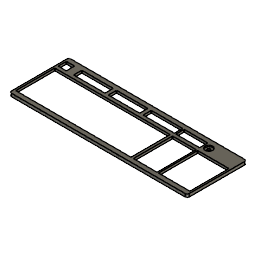
Top (Autodesk Fusion 360 design; units mm, degrees)
part number: 2026-01-27-17-33-11-118
Autodesk Fusion 360 part; units mm, degrees
(part 1 of 7)
sketch "Sketch1" plane through (0, 0, 0) normal (0, 0, 1) x (1, 0, 0)
  line L0 (-144.7637, -15.9426) -> (-144.7637, -18.7426)
  line L1 (-163.6637, -18.7426) -> (-163.6637, -15.9426)
  line L2 (-164.1637, -15.9426) -> (-164.1637, -18.7426)
  circle A0 centre (-169.0689, -18.2426) radius 2
  arc A1 (-107.101, -15.9426) -> (-108.601, -14.4426) centre (-108.601, -15.9426) ccw
  line L3 (-163.6635, 118.9832) -> (-163.6635, 116.1832)
  line L4 (-147.2637, -21.2426) -> (-161.6637, -21.2426)
  circle A2 centre (-169.0689, 118.4832) radius 2
  circle A3 centre (-169.0689, 118.4832) radius 1.7
  line L5 (-107.101, -15.9426) -> (-107.101, -18.7426)
  arc A4 (-144.7635, 116.1832) -> (-143.2635, 114.6832) centre (-143.2635, 116.1832) ccw
  arc A5 (-147.2637, -21.2426) -> (-144.7637, -18.7426) centre (-147.2637, -18.7426) ccw
  line L6 (-171.0689, 114.1832) -> (-165.6635, 114.1832)
  circle A6 centre (-151.9635, 117.5832) radius 1.7
  arc A7 (-164.1637, -18.7426) -> (-161.6637, -21.2426) centre (-161.6637, -18.7426) ccw
  line L7 (-161.6637, -20.7426) -> (-147.2637, -20.7426)
  circle A8 centre (-151.9635, 117.5832) radius 2
  line L8 (-165.6637, -13.9426) -> (-171.0689, -13.9426)
  circle A9 centre (-151.9637, -17.3426) radius 1.7
  line L9 (-165.6635, 114.6832) -> (-171.5689, 114.6832)
  arc A10 (-107.101, -18.7426) -> (-104.601, -21.2426) centre (-104.601, -18.7426) ccw
  arc A11 (-161.6635, 121.4832) -> (-164.1635, 118.9832) centre (-161.6635, 118.9832) ccw
  line L10 (-164.1635, 116.1832) -> (-164.1635, 118.9832)
  line L11 (-171.5689, -14.4426) -> (-165.6637, -14.4426)
  line L12 (-144.7635, 116.1832) -> (-144.7635, 118.9832)
  arc A12 (-169.0689, 123.4832) -> (-174.0689, 118.4832) centre (-169.0689, 118.4832) ccw
  arc A13 (-174.0689, -18.2426) -> (-169.0689, -23.2426) centre (-169.0689, -18.2426) ccw
  arc A14 (-165.6635, 114.6832) -> (-164.1635, 116.1832) centre (-165.6635, 116.1832) ccw
  circle A15 centre (-94.901, -17.3426) radius 1.7
  circle A16 centre (-94.901, -17.3426) radius 2
  circle A17 centre (-169.0689, -18.2426) radius 1.7
  line L13 (-106.601, -18.7426) -> (-106.601, -15.9426)
  line L14 (-145.2635, 118.9832) -> (-145.2635, 116.1832)
  line L15 (-143.2637, -14.4426) -> (-108.601, -14.4426)
  arc A18 (-144.7635, 118.9832) -> (-147.2635, 121.4832) centre (-147.2635, 118.9832) ccw
  line L16 (-82.701, -15.9426) -> (-82.701, -18.7426)
  arc A19 (-85.201, -21.2426) -> (-82.701, -18.7426) centre (-85.201, -18.7426) ccw
  circle A20 centre (42.9656, 118.4832) radius 1.7
  line L17 (-145.2637, -18.7426) -> (-145.2637, -15.9426)
  line L18 (28.798, 120.9832) -> (9.398, 120.9832)
  line L19 (-174.0689, 118.4832) -> (-174.0689, -18.2426)
  line L20 (-83.201, -18.7426) -> (-83.201, -15.9426)
  line L21 (-171.0689, 108.1832) -> (-171.0689, -7.9426)
  arc A21 (-82.701, 116.1832) -> (-81.201, 114.6832) centre (-81.201, 116.1832) ccw
  line L22 (9.398, 121.4832) -> (28.798, 121.4832)
  line L23 (30.798, 118.9832) -> (30.798, 116.1832)
  line L24 (-108.601, 114.6832) -> (-143.2635, 114.6832)
  arc A22 (-81.201, -14.4426) -> (-82.701, -15.9426) centre (-81.201, -15.9426) ccw
  circle A23 centre (-94.901, 117.5832) radius 2
  arc A24 (-82.701, 118.9832) -> (-85.201, 121.4832) centre (-85.201, 118.9832) ccw
  circle A25 centre (19.098, 117.5832) radius 2
  line L25 (-82.701, 116.1832) -> (-82.701, 118.9832)
  line L26 (-107.101, 116.1832) -> (-107.101, 118.9832)
  line L27 (31.298, 116.1832) -> (31.298, 118.9832)
  circle A26 centre (-94.901, 117.5832) radius 1.7
  arc A27 (5.398, 114.6832) -> (6.898, 116.1832) centre (5.398, 116.1832) ccw
  arc A28 (-164.1637, -15.9426) -> (-165.6637, -14.4426) centre (-165.6637, -15.9426) ccw
  arc A29 (31.298, 116.1832) -> (32.798, 114.6832) centre (32.798, 116.1832) ccw
  line L28 (-83.201, 118.9832) -> (-83.201, 116.1832)
  line L29 (6.898, 116.1832) -> (6.898, 118.9832)
  circle A30 centre (19.098, 117.5832) radius 1.7
  arc A31 (31.298, 118.9832) -> (28.798, 121.4832) centre (28.798, 118.9832) ccw
  arc A32 (9.398, 121.4832) -> (6.898, 118.9832) centre (9.398, 118.9832) ccw
  circle A33 centre (-151.9637, -17.3426) radius 2
  line L30 (-106.601, 118.9832) -> (-106.601, 116.1832)
  line L31 (7.398, 118.9832) -> (7.398, 116.1832)
  line L32 (-158.7961, 123.4832) -> (-169.0689, 123.4832)
  line L33 (-161.6635, 121.4832) -> (-147.2635, 121.4832)
  arc A34 (-108.601, 114.6832) -> (-107.101, 116.1832) centre (-108.601, 116.1832) ccw
  line L34 (-147.2635, 120.9832) -> (-161.6635, 120.9832)
  arc A35 (-143.2637, -14.4426) -> (-144.7637, -15.9426) centre (-143.2637, -15.9426) ccw
  arc A36 (-104.601, 121.4832) -> (-107.101, 118.9832) centre (-104.601, 118.9832) ccw
  circle A37 centre (19.098, -17.3426) radius 1.7
  line L35 (262.156, 114.6832) -> (262.156, -14.4426)
  line L36 (-104.601, 121.4832) -> (-85.201, 121.4832)
  line L37 (184.173, -15.9426) -> (184.173, -18.7426)
  line L38 (185.673, -14.4426) -> (222.567, -14.4426)
  line L39 (113.674, -14.4426) -> (158.273, -14.4426)
  line L40 (158.273, 114.6832) -> (113.674, 114.6832)
  line L41 (248.467, -15.9426) -> (248.467, -18.7426)
  line L42 (264.656, -18.2426) -> (264.656, 118.4832)
  circle A38 centre (19.098, -17.3426) radius 2
  line L43 (245.967, -21.2426) -> (226.567, -21.2426)
  line L44 (183.673, -18.7426) -> (183.673, -15.9426)
  circle A39 centre (171.973, -17.3426) radius 1.7
  line L45 (-85.201, 120.9832) -> (-104.601, 120.9832)
  arc A40 (224.067, -18.7426) -> (226.567, -21.2426) centre (226.567, -18.7426) ccw
  line L46 (-171.5689, 114.6832) -> (-171.5689, -14.4426)
  line L47 (261.656, 114.1832) -> (261.656, -13.9426)
  arc A41 (159.773, -15.9426) -> (158.273, -14.4426) centre (158.273, -15.9426) ccw
  line L48 (-169.0689, -23.2426) -> (42.9656, -23.2426)
  line L49 (6.898, -15.9426) -> (6.898, -18.7426)
  arc A42 (6.898, -15.9426) -> (5.398, -14.4426) centre (5.398, -15.9426) ccw
  line L50 (7.398, -18.7426) -> (7.398, -15.9426)
  line L51 (5.398, 114.6832) -> (-81.201, 114.6832)
  line L52 (9.398, -20.7426) -> (28.798, -20.7426)
  arc A43 (6.898, -18.7426) -> (9.398, -21.2426) centre (9.398, -18.7426) ccw
  line L53 (-81.201, -14.4426) -> (5.398, -14.4426)
  line L54 (28.798, -21.2426) -> (9.398, -21.2426)
  line L55 (-171.0689, -13.9426) -> (-171.0689, 114.1832)
  arc A44 (264.656, 118.4832) -> (259.656, 123.4832) centre (259.656, 118.4832) ccw
  line L56 (181.673, 120.9832) -> (162.273, 120.9832)
  line L57 (248.467, 118.9832) -> (248.467, 116.1832)
  circle A45 centre (259.656, -18.2426) radius 2
  line L58 (226.567, -20.7426) -> (245.967, -20.7426)
  arc A46 (159.773, -18.7426) -> (162.273, -21.2426) centre (162.273, -18.7426) ccw
  circle A47 centre (236.267, -17.3426) radius 1.7
  line L59 (181.673, -21.2426) -> (162.273, -21.2426)
  circle A48 centre (236.267, -17.3426) radius 2
  line L60 (160.273, -18.7426) -> (160.273, -15.9426)
  arc A49 (245.967, -21.2426) -> (248.467, -18.7426) centre (245.967, -18.7426) ccw
  arc A50 (224.067, -15.9426) -> (222.567, -14.4426) centre (222.567, -15.9426) ccw
  arc A51 (181.673, -21.2426) -> (184.173, -18.7426) centre (181.673, -18.7426) ccw
  line L61 (224.567, -18.7426) -> (224.567, -15.9426)
  line L62 (247.967, -18.7426) -> (247.967, -15.9426)
  line L63 (159.773, -15.9426) -> (159.773, -18.7426)
  arc A52 (259.656, -23.2426) -> (264.656, -18.2426) centre (259.656, -18.2426) ccw
  line L64 (224.067, -15.9426) -> (224.067, -18.7426)
  circle A53 centre (259.656, -18.2426) radius 1.7
  line L65 (-85.201, -21.2426) -> (-104.601, -21.2426)
  circle A54 centre (171.973, -17.3426) radius 2
  arc A55 (32.798, -14.4426) -> (31.298, -15.9426) centre (32.798, -15.9426) ccw
  line L66 (162.273, -20.7426) -> (181.673, -20.7426)
  line L67 (31.298, -15.9426) -> (31.298, -18.7426)
  circle A56 centre (42.9656, -18.2426) radius 1.7
  arc A57 (28.798, -21.2426) -> (31.298, -18.7426) centre (28.798, -18.7426) ccw
  arc A58 (249.967, -14.4426) -> (248.467, -15.9426) centre (249.967, -15.9426) ccw
  line L68 (30.798, -18.7426) -> (30.798, -15.9426)
  arc A59 (185.673, -14.4426) -> (184.173, -15.9426) centre (185.673, -15.9426) ccw
  line L69 (-104.601, -20.7426) -> (-85.201, -20.7426)
  line L70 (249.967, -14.4426) -> (262.156, -14.4426)
  circle A60 centre (99.974, -17.3426) radius 1.7
  circle A61 centre (99.974, 117.5832) radius 2
  line L71 (88.274, -18.7426) -> (88.274, -15.9426)
  line L72 (109.674, -21.2426) -> (90.274, -21.2426)
  line L73 (87.774, -15.9426) -> (87.774, -18.7426)
  line L74 (87.774, 116.1832) -> (87.774, 118.9832)
  line L75 (112.174, 116.1832) -> (112.174, 118.9832)
  arc A62 (109.674, -21.2426) -> (112.174, -18.7426) centre (109.674, -18.7426) ccw
  arc A63 (112.174, 118.9832) -> (109.674, 121.4832) centre (109.674, 118.9832) ccw
  line L76 (111.674, -18.7426) -> (111.674, -15.9426)
  line L77 (90.274, 121.4832) -> (109.674, 121.4832)
  arc A64 (87.774, -18.7426) -> (90.274, -21.2426) centre (90.274, -18.7426) ccw
  arc A65 (90.274, 121.4832) -> (87.774, 118.9832) centre (90.274, 118.9832) ccw
  circle A66 centre (99.974, 117.5832) radius 1.7
  line L78 (259.656, 123.4832) -> (-158.7961, 123.4832)
  arc A67 (113.674, -14.4426) -> (112.174, -15.9426) centre (113.674, -15.9426) ccw
  line L79 (111.674, 118.9832) -> (111.674, 116.1832)
  line L80 (90.274, -20.7426) -> (109.674, -20.7426)
  line L81 (109.674, 120.9832) -> (90.274, 120.9832)
  line L82 (86.274, 114.6832) -> (32.798, 114.6832)
  arc A68 (112.174, 116.1832) -> (113.674, 114.6832) centre (113.674, 116.1832) ccw
  arc A69 (86.274, 114.6832) -> (87.774, 116.1832) centre (86.274, 116.1832) ccw
  line L83 (88.274, 118.9832) -> (88.274, 116.1832)
  line L84 (112.174, -15.9426) -> (112.174, -18.7426)
  circle A70 centre (99.974, -17.3426) radius 2
  arc A71 (87.774, -15.9426) -> (86.274, -14.4426) centre (86.274, -15.9426) ccw
  circle A72 centre (236.267, 117.5832) radius 1.7
  arc A73 (226.567, 121.4832) -> (224.067, 118.9832) centre (226.567, 118.9832) ccw
  line L85 (245.967, 120.9832) -> (226.567, 120.9832)
  line L86 (262.156, 114.6832) -> (249.967, 114.6832)
  circle A74 centre (236.267, 117.5832) radius 2
  arc A75 (184.173, 116.1832) -> (185.673, 114.6832) centre (185.673, 116.1832) ccw
  line L87 (224.067, 116.1832) -> (224.067, 118.9832)
  line L88 (226.567, 121.4832) -> (245.967, 121.4832)
  line L89 (-169.0689, -23.2426) -> (259.656, -23.2426)
  arc A76 (222.567, 114.6832) -> (224.067, 116.1832) centre (222.567, 116.1832) ccw
  line L90 (262.156, -14.4426) -> (-171.5689, -14.4426)
  line L91 (32.798, -14.4426) -> (86.274, -14.4426)
  line L92 (261.656, -7.9426) -> (261.656, 108.1832)
  line L93 (159.773, 116.1832) -> (159.773, 118.9832)
  line L94 (160.273, 118.9832) -> (160.273, 116.1832)
  arc A77 (248.467, 116.1832) -> (249.967, 114.6832) centre (249.967, 116.1832) ccw
  circle A78 centre (259.656, 118.4832) radius 1.7
  line L95 (-171.5689, 114.6832) -> (262.156, 114.6832)
  circle A79 centre (259.656, 118.4832) radius 2
  arc A80 (248.467, 118.9832) -> (245.967, 121.4832) centre (245.967, 118.9832) ccw
  arc A81 (158.273, 114.6832) -> (159.773, 116.1832) centre (158.273, 116.1832) ccw
  arc A82 (184.173, 118.9832) -> (181.673, 121.4832) centre (181.673, 118.9832) ccw
  line L96 (222.567, 114.6832) -> (185.673, 114.6832)
  line L97 (247.967, 118.9832) -> (247.967, 116.1832)
  line L98 (224.567, 118.9832) -> (224.567, 116.1832)
  line L99 (184.173, 116.1832) -> (184.173, 118.9832)
  line L100 (162.273, 121.4832) -> (181.673, 121.4832)
  circle A83 centre (171.973, 117.5832) radius 1.7
  circle A84 centre (171.973, 117.5832) radius 2
  line L101 (183.673, 118.9832) -> (183.673, 116.1832)
  arc A85 (162.273, 121.4832) -> (159.773, 118.9832) centre (162.273, 118.9832) ccw
  line L102 (-154.9635, 117.5832) -> (-154.9635, 114.6832)
  line L103 (-148.9635, 117.5832) -> (-148.9635, 114.6832)
  arc A86 (-148.9635, 117.5832) -> (-154.9635, 117.5832) centre (-151.9635, 117.5832) ccw
  line L104 (-97.901, 117.5832) -> (-97.901, 114.6832)
  arc A87 (-91.901, 117.5832) -> (-97.901, 117.5832) centre (-94.901, 117.5832) ccw
  line L105 (-91.901, 117.5832) -> (-91.901, 114.6832)
  line L106 (16.098, 117.5832) -> (16.098, 114.6832)
  arc A88 (22.098, 117.5832) -> (16.098, 117.5832) centre (19.098, 117.5832) ccw
  line L107 (22.098, 117.5832) -> (22.098, 114.6832)
  line L108 (102.974, 117.5832) -> (102.974, 114.6832)
  arc A89 (102.974, 117.5832) -> (96.974, 117.5832) centre (99.974, 117.5832) ccw
  line L109 (96.974, 117.5832) -> (96.974, 114.6832)
  line L110 (174.973, 117.5832) -> (174.973, 114.6832)
  arc A90 (174.973, 117.5832) -> (168.973, 117.5832) centre (171.973, 117.5832) ccw
  line L111 (168.973, 117.5832) -> (168.973, 114.6832)
  line L112 (239.267, 117.5832) -> (239.267, 114.6832)
  arc A91 (239.267, 117.5832) -> (233.267, 117.5832) centre (236.267, 117.5832) ccw
  line L113 (233.267, 117.5832) -> (233.267, 114.6832)
  line L114 (239.267, -17.3426) -> (239.267, -14.4426)
  arc A92 (233.267, -17.3426) -> (239.267, -17.3426) centre (236.267, -17.3426) ccw
  line L115 (233.267, -17.3426) -> (233.267, -14.4426)
  arc A93 (168.973, -17.3426) -> (174.973, -17.3426) centre (171.973, -17.3426) ccw
  line L116 (174.973, -17.3426) -> (174.973, -14.4426)
  line L117 (168.973, -17.3426) -> (168.973, -14.4426)
  line L118 (102.974, -17.3426) -> (102.974, -14.4426)
  arc A94 (96.974, -17.3426) -> (102.974, -17.3426) centre (99.974, -17.3426) ccw
  line L119 (96.974, -17.3426) -> (96.974, -14.4426)
  line L120 (22.098, -17.3426) -> (22.098, -14.4426)
  arc A95 (16.098, -17.3426) -> (22.098, -17.3426) centre (19.098, -17.3426) ccw
  line L121 (16.098, -17.3426) -> (16.098, -14.4426)
  line L122 (-91.901, -17.3426) -> (-91.901, -14.4426)
  arc A96 (-97.901, -17.3426) -> (-91.901, -17.3426) centre (-94.901, -17.3426) ccw
  line L123 (-97.901, -17.3426) -> (-97.901, -14.4426)
  arc A97 (-154.9637, -17.3426) -> (-148.9637, -17.3426) centre (-151.9637, -17.3426) ccw
  line L124 (-148.9637, -17.3426) -> (-148.9637, -14.4426)
  line L125 (-154.9637, -17.3426) -> (-154.9637, -14.4426)
  circle A98 centre (42.9656, -18.2426) radius 2
  circle A99 centre (42.9656, 118.4832) radius 2
  dimension "d1" = 3
  dimension "d2" = 2.5
  dimension "d3" = 3
  dimension "d4" = 2.5
  dimension "d5" = 5
  dimension "d6" = 5
  dimension "d7" = 0.5
  dimension "d8" = 0.5
  dimension "d9" = 0.5
  dimension "d10" = 0.5
  dimension "d11" = 0.5
  dimension "d12" = 0.5
  dimension "d13" = 0.5
  dimension "d14" = 0.5
  dimension "d15" = 0.5
  dimension "d16" = 0.5
  dimension "d17" = 0.5
  dimension "d18" = 0.5
  dimension "d19" = 0.5
  dimension "d20" = 0.5
  dimension "d21" = 0.5
  dimension "d22" = 0.5
  dimension "d23" = 0.5
  dimension "d24" = 0.5
  dimension "d25" = 0.5
  dimension "d26" = 0.5
  dimension "d27" = 0.5
  dimension "d28" = 0.5
  dimension "d29" = 0.5
  dimension "d30" = 0.5
  dimension "d31" = 0.5
  dimension "d32" = 0.5
  dimension "d33" = 0.5
  dimension "d34" = 0.5
  dimension "d35" = 0.5
  dimension "d36" = 2.5
  dimension "d37" = 0.5
  dimension "d38" = 1.5
  dimension "d39" = 3.4
  dimension "d40" = 3.4
  dimension "d41" = 11.7
  dimension "d42" = 3.4
  dimension "d43" = 11.7
  dimension "d44" = 3.4
  dimension "d45" = 3.4
  dimension "d46" = 11.7
  dimension "d47" = 3.4
  dimension "d48" = 3.4
  dimension "d49" = 11.7
  dimension "d50" = 3.4
  dimension "d51" = 3.4
  dimension "d52" = 11.7
  dimension "d53" = 3.4
  dimension "d54" = 3.4
  dimension "d55" = 3.4
  dimension "d56" = 11.7
  dimension "d57" = 3.4
  dimension "d58" = 3.4
  dimension "d59" = 11.7
  dimension "d60" = 3.4
  dimension "d61" = 11.7
  dimension "d62" = 3.4
  dimension "d63" = 3.4
  dimension "d64" = 3.4
  dimension "d65" = 11.7
  dimension "d66" = 3.4
  dimension "d67" = 3.4
  dimension "d68" = 11.7
  dimension "d69" = 3.4
  dimension "d70" = 11.7
  dimension "d71" = 3.4
  dimension "d72" = 3.4
  dimension "d73" = 11.7
  dimension "d74" = 3.4
  dimension "d75" = 4
  dimension "d76" = 4
  dimension "d77" = 4
  dimension "d78" = 4
  dimension "d79" = 4
  dimension "d80" = 4
  dimension "d81" = 4
  dimension "d82" = 4
  dimension "d83" = 4
  dimension "d84" = 4
  dimension "d85" = 4
  dimension "d86" = 4
  dimension "d87" = 3.4
  dimension "d88" = 5
  dimension "d89" = 5
  dimension "d90" = 3.4
  dimension "d91" = 5
  dimension "d92" = 5
  dimension "d93" = 3.4
  dimension "d94" = 3.4
  dimension "d95" = 5
  dimension "d96" = 5
  dimension "d97" = 5
  dimension "d98" = 5
  dimension "d99" = 212.0345
  dimension "d100" = 3.4
  dimension "d101" = 3.4
  dimension "d102" = 5
  dimension "d103" = 5
  dimension "d104" = 4
  dimension "d105" = 4
  dimension "d106" = 4
  dimension "d107" = 4
  dimension "d112" = 6
  dimension "d122" = 3
  dimension "d123" = 3
  dimension "d124" = 6
  dimension "d125" = 6
  dimension "d126" = 6
  dimension "d127" = 6
  dimension "d128" = 6
  dimension "d129" = 6
  dimension "d130" = 6
  dimension "d131" = 6
  dimension "d132" = 6
  dimension "d133" = 6
  dimension "d134" = 6
  dimension "d224" = 4
  dimension "d225" = 4
  constraint vertical L19
  constraint perpendicular L21 L89
  constraint vertical L42
  constraint horizontal L78
  constraint parallel L32 L78
  constraint tangent A13 L89
  constraint tangent A13 L19
  constraint tangent A12 L19
  constraint tangent A12 L32
  constraint equal A12 A13
  constraint tangent L42 A44
  constraint tangent A44 L78
  constraint equal A13 A44
  constraint tangent A52 L89
  constraint tangent L42 A52
  constraint parallel L77 L78
  constraint parallel L24 L33
  constraint parallel L21 L46
  constraint perpendicular L11 L46
  constraint parallel L43 L89
  constraint vertical L2
  constraint perpendicular L0 L4
  constraint perpendicular L5 L65
  constraint perpendicular L16 L65
  constraint perpendicular L49 L54
  constraint perpendicular L54 L67
  constraint perpendicular L72 L73
  constraint perpendicular L72 L84
  constraint perpendicular L59 L63
  constraint perpendicular L37 L59
  constraint perpendicular L43 L64
  constraint perpendicular L41 L43
  constraint perpendicular L35 L86
  constraint collinear L4 L65
  constraint collinear L54 L65
  constraint collinear L54 L72
  constraint collinear L59 L72
  constraint collinear L43 L59
  constraint perpendicular L57 L86
  constraint perpendicular L87 L88
  constraint perpendicular L99 L100
  constraint perpendicular L93 L100
  constraint perpendicular L75 L77
  constraint perpendicular L74 L77
  constraint perpendicular L22 L27
  constraint perpendicular L22 L29
  constraint perpendicular L25 L36
  constraint perpendicular L26 L36
  constraint perpendicular L12 L33
  constraint perpendicular L10 L33
  constraint collinear L88 L100
  constraint collinear L77 L100
  constraint collinear L22 L77
  constraint collinear L22 L36
  constraint collinear L33 L36
  constraint collinear L9 L24
  constraint collinear L24 L51
  constraint collinear L51 L82
  constraint collinear L40 L82
  constraint collinear L40 L96
  constraint collinear L86 L96
  constraint collinear L38 L70
  constraint collinear L38 L39
  constraint collinear L39 L91
  constraint collinear L53 L91
  constraint collinear L15 L53
  constraint collinear L11 L15
  constraint tangent L2 A7
  constraint tangent L4 A7
  constraint tangent L0 A5
  constraint tangent L4 A5
  constraint equal A5 A7
  constraint tangent L5 A10
  constraint tangent A10 L65
  constraint equal A7 A10
  constraint tangent L16 A19
  constraint tangent A19 L65
  constraint equal A7 A19
  constraint tangent L49 A43
  constraint tangent A43 L54
  constraint equal A7 A43
  constraint tangent L67 A57
  constraint tangent L54 A57
  constraint equal A7 A57
  constraint tangent L73 A64
  constraint tangent L72 A64
  constraint equal A7 A64
  constraint tangent A62 L84
  constraint tangent L72 A62
  constraint equal A7 A62
  constraint tangent A46 L63
  constraint tangent A46 L59
  constraint equal A7 A46
  constraint tangent L37 A51
  constraint tangent L59 A51
  constraint equal A7 A51
  constraint tangent A40 L64
  constraint tangent L43 A40
  constraint equal A7 A40
  constraint tangent L41 A49
  constraint tangent L43 A49
  constraint equal A7 A49
  constraint tangent L57 A80
  constraint tangent L88 A80
  constraint equal A7 A80
  constraint tangent A73 L87
  constraint tangent A73 L88
  constraint equal A7 A73
  constraint tangent A82 L99
  constraint tangent A82 L100
  constraint equal A7 A82
  constraint tangent L93 A85
  constraint tangent L100 A85
  constraint equal A7 A85
  constraint tangent L75 A63
  constraint tangent A63 L77
  constraint equal A7 A63
  constraint tangent L74 A65
  constraint tangent L77 A65
  constraint equal A7 A65
  constraint tangent L27 A31
  constraint tangent L22 A31
  constraint equal A7 A31
  constraint tangent L29 A32
  constraint tangent L22 A32
  constraint equal A7 A32
  constraint tangent A24 L25
  constraint tangent A24 L36
  constraint equal A7 A24
  constraint tangent L26 A36
  constraint tangent A36 L36
  constraint equal A7 A36
  constraint tangent L12 A18
  constraint tangent A18 L33
  constraint equal A7 A18
  constraint tangent A11 L10
  constraint tangent A11 L33
  constraint equal A7 A11
  constraint tangent L2 A28
  constraint tangent L11 A28
  constraint tangent L0 A35
  constraint tangent L15 A35
  constraint equal A28 A35
  constraint tangent A1 L5
  constraint tangent A1 L15
  constraint equal A1 A28
  constraint tangent L16 A22
  constraint tangent A22 L53
  constraint equal A22 A28
  constraint tangent L49 A42
  constraint tangent A42 L53
  constraint equal A28 A42
  constraint tangent A55 L67
  constraint tangent A55 L91
  constraint equal A28 A55
  constraint tangent L73 A71
  constraint tangent A71 L91
  constraint equal A28 A71
  constraint tangent A67 L84
  constraint tangent L39 A67
  constraint equal A28 A67
  constraint tangent A41 L63
  constraint tangent L39 A41
  constraint equal A28 A41
  constraint tangent L37 A59
  constraint tangent L38 A59
  constraint equal A28 A59
  constraint tangent A50 L64
  constraint tangent L38 A50
  constraint equal A28 A50
  constraint tangent L41 A58
  constraint tangent A58 L70
  constraint equal A28 A58
  constraint tangent L57 A77
  constraint tangent L86 A77
  constraint equal A28 A77
  constraint tangent L87 A76
  constraint tangent A76 L96
  constraint equal A28 A76
  constraint tangent A75 L99
  constraint tangent A75 L96
  constraint equal A28 A75
  constraint tangent L93 A81
  constraint tangent L40 A81
  constraint equal A28 A81
  constraint tangent L75 A68
  constraint tangent L40 A68
  constraint equal A28 A68
  constraint tangent L74 A69
  constraint tangent L82 A69
  constraint equal A28 A69
  constraint tangent L27 A29
  constraint tangent A29 L82
  constraint equal A28 A29
  constraint tangent A27 L29
  constraint tangent A27 L51
  constraint equal A27 A28
  constraint tangent A21 L25
  constraint tangent A21 L51
  constraint equal A21 A28
  constraint tangent L26 A34
  constraint tangent L24 A34
  constraint equal A28 A34
  constraint tangent A4 L12
  constraint tangent A4 L24
  constraint equal A4 A28
  constraint tangent L10 A14
  constraint tangent L9 A14
  constraint equal A14 A28
  constraint concentric A9 A33
  constraint concentric A15 A16
  constraint concentric A37 A38
  constraint concentric A60 A70
  constraint concentric A39 A54
  constraint concentric A47 A48
  constraint concentric A72 A74
  constraint concentric A83 A84
  constraint concentric A61 A66
  constraint concentric A25 A30
  constraint concentric A23 A26
  constraint concentric A6 A8
  constraint parallel L48 L89
  constraint concentric A0 A17
  constraint concentric A2 A3
  constraint concentric A44 A79
  constraint concentric A45 A53
  constraint concentric A6 A86
  constraint coincident L95 L102.end
  constraint perpendicular L95 L102
  constraint coincident L95 L103.end
  constraint perpendicular L95 L103
  constraint concentric A56 A98
  constraint concentric A20 A99
  measures "d1" distance of L19 L21
  measures "d2" distance of L58 L89
  measures "d3" distance of L42 L47
  measures "d4" distance of L32 L34
  measures "d5" radius of A13
  measures "d6" radius of A52
  measures "d7" distance of L85 L88
  measures "d8" distance of L6 L9
  measures "d9" distance of L46 L55
  measures "d10" distance of L4 L7
  measures "d11" distance of L1 L2
  measures "d12" distance of L0 L17
  measures "d13" distance of L5 L13
  measures "d14" distance of L16 L20
  measures "d15" distance of L49 L50
  measures "d16" distance of L67 L68
  measures "d17" distance of L71 L73
  measures "d18" distance of L76 L84
  measures "d19" distance of L60 L63
  measures "d20" distance of L37 L44
  measures "d21" distance of L61 L64
  measures "d22" distance of L41 L62
  measures "d23" distance of L35 L92
  measures "d24" distance of L3 L10
  measures "d25" distance of L12 L14
  measures "d26" distance of L26 L30
  measures "d27" distance of L25 L28
  measures "d28" distance of L29 L31
  measures "d29" distance of L23 L27
  measures "d30" distance of L74 L83
  measures "d31" distance of L75 L79
  measures "d32" distance of L93 L94
  measures "d33" distance of L99 L101
  measures "d34" distance of L87 L98
  measures "d35" distance of L57 L97
  measures "d36" radius of A7
  measures "d37" distance of L8 L11
  measures "d38" radius of A28
  measures "d39" diameter of A6
  measures "d40" distance of A6.centre L34
  measures "d41" distance of A6.centre L3
  measures "d42" diameter of A26
  measures "d43" distance of A23.centre L30
  measures "d44" distance of A23.centre L45
  measures "d45" diameter of A30
  measures "d46" distance of A25.centre L31
  measures "d47" distance of A25.centre L18
  measures "d48" diameter of A66
  measures "d49" distance of A61.centre L83
  measures "d50" distance of A61.centre L81
  measures "d51" diameter of A83
  measures "d52" distance of A83.centre L94
  measures "d53" distance of A83.centre L56
  measures "d54" diameter of A72
  measures "d55" distance of A72.centre L85
  measures "d56" distance of A72.centre L98
  measures "d57" diameter of A47
  measures "d58" distance of A47.centre L58
  measures "d59" distance of A47.centre L61
  measures "d60" diameter of A39
  measures "d61" distance of A39.centre L60
  measures "d62" distance of A39.centre L66
  measures "d63" diameter of A60
  measures "d64" distance of A60.centre L80
  measures "d65" distance of A60.centre L71
  measures "d66" diameter of A37
  measures "d67" distance of A37.centre L52
  measures "d68" distance of A37.centre L50
  measures "d69" diameter of A15
  measures "d70" distance of A15.centre L13
  measures "d71" distance of A15.centre L69
  measures "d72" diameter of A9
  measures "d73" distance of A9.centre L1
  measures "d74" distance of A9.centre L7
  measures "d75" diameter of A33
  measures "d76" diameter of A16
  measures "d77" diameter of A38
  measures "d78" diameter of A70
  measures "d79" diameter of A54
  measures "d80" diameter of A48
  measures "d81" diameter of A74
  measures "d82" diameter of A84
  measures "d83" diameter of A61
  measures "d84" diameter of A25
  measures "d85" diameter of A23
  measures "d86" diameter of A8
  measures "d87" diameter of A78
  measures "d88" distance of A44.centre L42
  measures "d89" distance of A44.centre L78
  measures "d90" diameter of A53
  measures "d91" distance of A45.centre L42
  measures "d92" distance of A45.centre L89
  measures "d93" diameter of A17
  measures "d94" diameter of A3
  measures "d95" distance of A2.centre L32
  measures "d96" distance of A2.centre L19
  measures "d97" distance of A0.centre L19
  measures "d98" distance of A0.centre L89
  measures "d99" distance of A13.end L48.end
  measures "d100" diameter of A56
  measures "d101" diameter of A20
  measures "d102" distance of A20.centre L78
  measures "d103" distance of A56.centre L89
  measures "d104" diameter of A0
  measures "d105" diameter of A2
  measures "d106" diameter of A79
  measures "d107" diameter of A45
  measures "d112" diameter of A86
  measures "d122" distance of A6.centre L102
  measures "d123" distance of A6.centre L103
  measures "d124" diameter of A87
  measures "d125" diameter of A88
  measures "d126" diameter of A89
  measures "d127" diameter of A90
  measures "d128" diameter of A91
  measures "d129" diameter of A92
  measures "d130" diameter of A93
  measures "d131" diameter of A94
  measures "d132" diameter of A95
  measures "d133" diameter of A96
  measures "d134" diameter of A97
  measures "d224" diameter of A98
  measures "d225" diameter of A99
sketch "Sketch2" plane through (0, 0, 0) normal (0, 0, 1) x (1, 0, 0)
  line L0 (98.973, 37.709) -> (98.973, 38.5083)
  line L1 (110.974, 38.5083) -> (110.974, 37.709)
  line L2 (111.423, 35.2589) -> (111.423, 31.9583)
  line L3 (107.274, 38.5083) -> (107.274, 36.984)
  line L4 (102.673, 38.5083) -> (102.673, 36.984)
  line L5 (107.874, 37.709) -> (107.874, 38.5083)
  line L6 (86.274, -13.9426) -> (32.798, -13.9426)
  line L7 (110.503, 35.2589) -> (110.503, 36.984)
  line L8 (98.204, 36.984) -> (102.673, 36.984)
  line L9 (110.503, 36.984) -> (110.503, 35.2589)
  line L10 (97.974, 38.5083) -> (98.973, 38.5083)
  line L11 (107.274, 36.984) -> (110.503, 36.984)
  line L12 (97.224, 35.2589) -> (97.224, 31.9583)
  line L13 (110.974, 37.709) -> (110.974, 38.5083)
  line L14 (111.973, 38.5083) -> (110.974, 38.5083)
  line L15 (97.224, 35.2589) -> (98.204, 35.2589)
  line L16 (102.073, 37.709) -> (98.973, 37.709)
  line L17 (110.974, 37.709) -> (107.874, 37.709)
  line L18 (98.204, 36.984) -> (98.204, 35.2589)
  line L19 (43.205, 81.084) -> (57.206, 81.084)
  line L20 (57.206, 81.084) -> (43.205, 81.084)
  line L21 (32.798, 114.1832) -> (86.274, 114.1832)
  line L22 (47.681, 48.0333) -> (33.68, 48.0333)
  line L23 (38.442, 42.984) -> (52.442, 42.984)
  line L24 (33.68, 62.034) -> (47.681, 62.034)
  line L25 (142.417, 22.9336) -> (143.217, 22.9336)
  line L26 (143.217, 22.9336) -> (143.217, 23.934)
  line L27 (142.417, 19.8345) -> (143.217, 19.8345)
  line L28 (111.423, 35.2589) -> (110.503, 35.2589)
  line L29 (98.973, 38.5083) -> (98.973, 37.709)
  line L30 (102.073, 38.5083) -> (102.073, 37.709)
  line L31 (110.503, 36.984) -> (107.274, 36.984)
  line L32 (142.417, 19.8345) -> (142.417, 22.9336)
  line L33 (143.217, 22.9336) -> (142.417, 22.9336)
  line L34 (143.217, 19.8345) -> (142.417, 19.8345)
  line L35 (143.217, 19.8345) -> (143.217, 14.0343)
  line L36 (142.417, 22.9336) -> (142.417, 19.8345)
  line L37 (143.217, 23.934) -> (143.217, 22.9336)
  line L38 (143.217, 14.0343) -> (143.217, 19.8345)
  line L39 (110.503, 30.2332) -> (110.503, 31.9583)
  line L40 (111.423, 31.9583) -> (110.503, 31.9583)
  line L41 (107.274, 29.4092) -> (104.474, 29.4092)
  line L42 (104.474, 29.4092) -> (104.474, 30.2332)
  line L43 (98.204, 31.9583) -> (98.204, 30.2332)
  line L44 (110.503, 31.9583) -> (110.503, 30.2332)
  line L45 (98.204, 30.2332) -> (98.204, 31.9583)
  line L46 (104.474, 29.4092) -> (107.274, 29.4092)
  line L47 (110.503, 30.2332) -> (107.274, 30.2332)
  line L48 (107.274, 30.2332) -> (107.274, 29.4092)
  line L49 (98.204, 30.2332) -> (104.474, 30.2332)
  line L50 (104.474, 30.2332) -> (104.474, 29.4092)
  line L51 (105.961, 22.4637) -> (104.237, 22.4637)
  line L52 (104.237, 23.3844) -> (100.937, 23.3844)
  line L53 (97.687, 22.9336) -> (97.687, 23.934)
  line L54 (98.486, 22.9336) -> (98.486, 19.8345)
  line L55 (111.423, 31.9583) -> (111.423, 35.2589)
  line L56 (102.073, 37.709) -> (102.073, 38.5083)
  line L57 (102.673, 38.5083) -> (102.073, 38.5083)
  line L58 (97.224, 31.9583) -> (97.224, 35.2589)
  line L59 (110.503, 35.2589) -> (111.423, 35.2589)
  line L60 (107.274, 36.984) -> (107.274, 38.5083)
  line L61 (98.973, 37.709) -> (102.073, 37.709)
  line L62 (98.204, 35.2589) -> (98.204, 36.984)
  line L63 (107.874, 38.5083) -> (107.874, 37.709)
  line L64 (107.874, 37.709) -> (110.974, 37.709)
  line L65 (102.673, 36.984) -> (98.204, 36.984)
  line L66 (98.204, 35.2589) -> (97.224, 35.2589)
  line L67 (102.673, 36.984) -> (102.673, 38.5083)
  line L68 (107.274, 38.5083) -> (107.874, 38.5083)
  line L69 (98.973, 38.5083) -> (97.974, 38.5083)
  line L70 (107.874, 38.5083) -> (107.274, 38.5083)
  line L71 (110.974, 38.5083) -> (111.973, 38.5083)
  line L72 (97.974, 38.5083) -> (97.974, 52.509)
  line L73 (102.073, 38.5083) -> (102.673, 38.5083)
  line L74 (111.973, 38.5083) -> (111.973, 52.509)
  line L75 (97.974, 52.509) -> (97.974, 38.5083)
  line L76 (111.973, 52.509) -> (111.973, 38.5083)
  line L77 (110.503, 31.9583) -> (111.423, 31.9583)
  line L78 (104.474, 30.2332) -> (98.204, 30.2332)
  line L79 (97.224, 31.9583) -> (98.204, 31.9583)
  line L80 (107.274, 30.2332) -> (110.503, 30.2332)
  line L81 (98.204, 31.9583) -> (97.224, 31.9583)
  line L82 (107.274, 29.4092) -> (107.274, 30.2332)
  line L83 (138.968, 3.8837) -> (138.968, 0.7845)
  line L84 (143.217, 3.8837) -> (142.417, 3.8837)
  line L85 (142.417, 14.0343) -> (142.417, 10.9337)
  line L86 (124.167, 3.8837) -> (123.367, 3.8837)
  line L87 (143.217, 9.9333) -> (143.217, 10.9337)
  line L88 (124.167, 3.8837) -> (124.167, 4.8841)
  line L89 (99.211, 19.2336) -> (99.211, 22.4637)
  line L90 (100.937, 23.3844) -> (100.937, 22.4637)
  line L91 (100.937, 22.4637) -> (99.211, 22.4637)
  line L92 (104.237, 23.3844) -> (104.237, 22.4637)
  line L93 (106.786, 19.2336) -> (106.786, 16.4335)
  line L94 (97.687, 19.2336) -> (99.211, 19.2336)
  line L95 (97.687, 23.934) -> (97.687, 22.9336)
  line L96 (104.237, 22.4637) -> (104.237, 23.3844)
  line L97 (97.687, 19.8345) -> (98.486, 19.8345)
  line L98 (97.687, 19.8345) -> (97.687, 19.2336)
  line L99 (98.486, 19.8345) -> (97.687, 19.8345)
  line L100 (100.937, 23.3844) -> (104.237, 23.3844)
  line L101 (99.211, 19.2336) -> (97.687, 19.2336)
  line L102 (97.687, 22.9336) -> (98.486, 22.9336)
  line L103 (105.961, 16.4335) -> (106.786, 16.4335)
  line L104 (98.486, 22.9336) -> (97.687, 22.9336)
  line L105 (106.786, 19.2336) -> (105.961, 19.2336)
  line L106 (105.961, 19.2336) -> (106.786, 19.2336)
  line L107 (105.961, 19.2336) -> (105.961, 22.4637)
  line L108 (106.786, 16.4335) -> (106.786, 19.2336)
  line L109 (100.937, 22.4637) -> (100.937, 23.3844)
  line L110 (99.211, 22.4637) -> (100.937, 22.4637)
  line L111 (97.687, 19.2336) -> (97.687, 19.8345)
  line L112 (99.211, 22.4637) -> (99.211, 19.2336)
  line L113 (98.486, 19.8345) -> (98.486, 22.9336)
  line L114 (106.786, 16.4335) -> (105.961, 16.4335)
  line L115 (105.961, 22.4637) -> (105.961, 19.2336)
  line L116 (104.237, 22.4637) -> (105.961, 22.4637)
  line L117 (143.217, 14.0343) -> (142.417, 14.0343)
  line L118 (123.367, 3.8837) -> (124.167, 3.8837)
  line L119 (143.217, 10.9337) -> (142.417, 10.9337)
  line L120 (138.968, 0.7845) -> (138.968, 3.8837)
  line L121 (142.417, 0.7845) -> (142.417, 3.8837)
  line L122 (138.167, 4.8841) -> (138.167, 3.8837)
  line L123 (142.417, 14.0343) -> (143.217, 14.0343)
  line L124 (138.167, 3.8837) -> (138.167, 4.8841)
  line L125 (138.167, 4.8841) -> (124.167, 4.8841)
  line L126 (142.417, 10.9337) -> (143.217, 10.9337)
  line L127 (138.167, 3.8837) -> (138.968, 3.8837)
  line L128 (143.217, 10.9337) -> (143.217, 9.9333)
  line L129 (143.217, 3.8837) -> (143.217, 4.8841)
  line L130 (123.367, 0.7845) -> (123.367, 3.8837)
  line L131 (138.968, 3.8837) -> (138.167, 3.8837)
  line L132 (124.167, 4.8841) -> (124.167, 3.8837)
  line L133 (124.167, 4.8841) -> (138.167, 4.8841)
  line L134 (142.417, 3.8837) -> (142.417, 0.7845)
  line L135 (142.417, 10.9337) -> (142.417, 14.0343)
  line L136 (143.217, 4.8841) -> (143.217, 3.8837)
  line L137 (123.367, 3.8837) -> (123.367, 0.7845)
  line L138 (142.417, 3.8837) -> (143.217, 3.8837)
  line L139 (97.687, 10.9337) -> (97.687, 9.9333)
  line L140 (98.486, 10.9337) -> (97.687, 10.9337)
  line L141 (99.211, 10.1634) -> (99.211, 14.6338)
  line L142 (98.486, 14.0343) -> (98.486, 10.9337)
  line L143 (105.961, 10.1634) -> (105.961, 16.4335)
  line L144 (97.687, 14.6338) -> (97.687, 14.0343)
  line L145 (97.687, 14.0343) -> (97.687, 14.6338)
  line L146 (104.237, 10.1634) -> (104.237, 9.1836)
  line L147 (105.961, 10.1634) -> (104.237, 10.1634)
  line L148 (105.961, 16.4335) -> (105.961, 10.1634)
  line L149 (104.237, 9.1836) -> (100.937, 9.1836)
  line L150 (99.211, 10.1634) -> (100.937, 10.1634)
  line L151 (104.237, 9.1836) -> (104.237, 10.1634)
  line L152 (100.937, 9.1836) -> (104.237, 9.1836)
  line L153 (99.211, 14.6338) -> (99.211, 10.1634)
  line L154 (97.687, 14.0343) -> (98.486, 14.0343)
  line L155 (123.367, -5.0157) -> (124.167, -5.0157)
  line L156 (138.968, 0.7845) -> (138.167, 0.7845)
  line L157 (143.217, -9.1167) -> (143.217, -8.1163)
  line L158 (143.217, 0.7845) -> (143.217, -5.0157)
  line L159 (124.167, -8.1163) -> (123.367, -8.1163)
  line L160 (143.217, -5.0157) -> (143.217, 0.7845)
  line L161 (138.167, -8.1163) -> (138.167, -9.1167)
  line L162 (123.367, 0.7845) -> (124.167, 0.7845)
  line L163 (138.167, -5.0157) -> (138.167, 0.7845)
  line L164 (138.968, -8.1163) -> (138.968, -5.0157)
  line L165 (124.167, -9.1167) -> (124.167, -8.1163)
  line L166 (142.417, -5.0157) -> (142.417, -8.1163)
  line L167 (124.167, -9.1167) -> (138.167, -9.1167)
  line L168 (124.167, -5.0157) -> (124.167, 0.7845)
  line L169 (138.167, -9.1167) -> (124.167, -9.1167)
  line L170 (138.167, -9.1167) -> (138.167, -8.1163)
  line L171 (124.167, 0.7845) -> (124.167, -5.0157)
  line L172 (124.167, 0.7845) -> (123.367, 0.7845)
  line L173 (138.167, -8.1163) -> (138.968, -8.1163)
  line L174 (123.367, -5.0157) -> (123.367, -8.1163)
  line L175 (123.367, -8.1163) -> (124.167, -8.1163)
  line L176 (142.417, -8.1163) -> (143.217, -8.1163)
  line L177 (138.167, -5.0157) -> (138.968, -5.0157)
  line L178 (138.968, -5.0157) -> (138.167, -5.0157)
  line L179 (142.417, 0.7845) -> (143.217, 0.7845)
  line L180 (143.217, -8.1163) -> (142.417, -8.1163)
  line L181 (138.968, -5.0157) -> (138.968, -8.1163)
  line L182 (142.417, -5.0157) -> (143.217, -5.0157)
  line L183 (123.367, -8.1163) -> (123.367, -5.0157)
  line L184 (143.217, 0.7845) -> (142.417, 0.7845)
  line L185 (143.217, -5.0157) -> (142.417, -5.0157)
  line L186 (138.167, 0.7845) -> (138.968, 0.7845)
  line L187 (138.167, 0.7845) -> (138.167, -5.0157)
  line L188 (143.217, -8.1163) -> (143.217, -9.1167)
  line L189 (138.968, -8.1163) -> (138.167, -8.1163)
  line L190 (142.417, -8.1163) -> (142.417, -5.0157)
  line L191 (124.167, -8.1163) -> (124.167, -9.1167)
  line L192 (124.167, -5.0157) -> (123.367, -5.0157)
  line L193 (98.486, 14.0343) -> (97.687, 14.0343)
  line L194 (97.687, 14.6338) -> (99.211, 14.6338)
  line L195 (104.237, 10.1634) -> (105.961, 10.1634)
  line L196 (98.486, 10.9337) -> (98.486, 14.0343)
  line L197 (97.173, -8.1163) -> (97.974, -8.1163)
  line L198 (111.973, -9.1167) -> (111.973, -8.1163)
  line L199 (112.774, -8.1163) -> (111.973, -8.1163)
  line L200 (112.774, -8.1163) -> (112.774, -5.0157)
  line L201 (97.974, -8.1163) -> (97.974, -9.1167)
  line L202 (97.974, -5.0157) -> (97.173, -5.0157)
  line L203 (111.973, 0.7845) -> (111.973, -5.0157)
  line L204 (111.973, -8.1163) -> (112.774, -8.1163)
  line L205 (111.674, -18.7426) -> (111.674, -15.9426)
  line L206 (97.974, -9.1167) -> (111.973, -9.1167)
  line L207 (90.274, -20.7426) -> (109.674, -20.7426)
  line L208 (97.974, -8.1163) -> (97.173, -8.1163)
  line L209 (112.774, -5.0157) -> (111.973, -5.0157)
  line L210 (97.173, -8.1163) -> (97.173, -5.0157)
  line L211 (97.173, -5.0157) -> (97.974, -5.0157)
  line L212 (97.974, -5.0157) -> (97.974, 0.7845)
  line L213 (112.774, -5.0157) -> (112.774, -8.1163)
  line L214 (97.974, 0.7845) -> (97.974, -5.0157)
  line L215 (99.211, 14.6338) -> (97.687, 14.6338)
  line L216 (97.687, 9.9333) -> (97.687, 10.9337)
  line L217 (97.687, 10.9337) -> (98.486, 10.9337)
  line L218 (100.937, 10.1634) -> (100.937, 9.1836)
  line L219 (100.937, 9.1836) -> (100.937, 10.1634)
  line L220 (100.937, 10.1634) -> (99.211, 10.1634)
  line L221 (112.774, 0.7845) -> (112.774, 3.8837)
  line L222 (112.774, 3.8837) -> (112.774, 0.7845)
  line L223 (97.974, 4.8841) -> (97.974, 3.8837)
  line L224 (97.974, 3.8837) -> (97.173, 3.8837)
  line L225 (112.774, 3.8837) -> (111.973, 3.8837)
  line L226 (111.973, 3.8837) -> (112.774, 3.8837)
  line L227 (97.974, 0.7845) -> (97.173, 0.7845)
  line L228 (97.974, 3.8837) -> (97.974, 4.8841)
  line L229 (111.973, 4.8841) -> (97.974, 4.8841)
  line L230 (111.973, 0.7845) -> (112.774, 0.7845)
  line L231 (97.173, 3.8837) -> (97.974, 3.8837)
  line L232 (97.974, 4.8841) -> (111.973, 4.8841)
  line L233 (111.973, 4.8841) -> (111.973, 3.8837)
  line L234 (112.774, 0.7845) -> (111.973, 0.7845)
  line L235 (97.173, 0.7845) -> (97.173, 3.8837)
  line L236 (97.173, 0.7845) -> (97.974, 0.7845)
  line L237 (111.973, 3.8837) -> (111.973, 4.8841)
  line L238 (97.173, 3.8837) -> (97.173, 0.7845)
  line L239 (111.973, -5.0157) -> (112.774, -5.0157)
  line L240 (111.973, -8.1163) -> (111.973, -9.1167)
  circle A0 centre (99.974, -17.3426) radius 1.7
  arc A1 (109.674, -20.7426) -> (111.674, -18.7426) centre (109.674, -18.7426) ccw
  circle A2 centre (99.974, -17.3426) radius 1.7
  line L241 (111.973, -5.0157) -> (111.973, 0.7845)
  line L242 (99.574, -20.7426) -> (100.374, -20.7426)
  line L243 (111.973, -9.1167) -> (97.974, -9.1167)
  line L244 (97.173, -5.0157) -> (97.173, -8.1163)
  arc A3 (113.674, -13.9426) -> (111.674, -15.9426) centre (113.674, -15.9426) ccw
  line L245 (97.974, -9.1167) -> (97.974, -8.1163)
  line L246 (76.542, 33.0844) -> (76.542, 38.8844)
  line L247 (90.542, 42.984) -> (90.542, 41.9836)
  line L248 (75.742, 29.9838) -> (75.742, 33.0844)
  line L249 (75.742, 33.0844) -> (75.742, 29.9838)
  line L250 (75.742, 41.9836) -> (75.742, 38.8844)
  line L251 (75.742, 29.9838) -> (76.542, 29.9838)
  line L252 (76.542, 41.9836) -> (76.542, 42.984)
  line L253 (75.742, 38.8844) -> (76.542, 38.8844)
  line L254 (90.542, 42.984) -> (76.542, 42.984)
  line L255 (90.542, 33.0844) -> (90.542, 38.8844)
  line L256 (76.542, 28.9833) -> (90.542, 28.9833)
  line L257 (76.542, 41.9836) -> (75.742, 41.9836)
  line L258 (76.542, 42.984) -> (90.542, 42.984)
  line L259 (90.542, 28.9833) -> (76.542, 28.9833)
  line L260 (80.435, 23.3844) -> (77.137, 23.3844)
  line L261 (83.685, 22.9336) -> (83.685, 23.934)
  line L262 (82.887, 19.8345) -> (82.887, 22.9336)
  line L263 (75.411, 16.4335) -> (74.587, 16.4335)
  line L264 (90.542, 38.8844) -> (90.542, 33.0844)
  line L265 (91.343, 41.9836) -> (90.542, 41.9836)
  line L266 (91.343, 33.0844) -> (90.542, 33.0844)
  line L267 (90.542, 38.8844) -> (91.343, 38.8844)
  line L268 (90.542, 41.9836) -> (91.343, 41.9836)
  line L269 (90.542, 33.0844) -> (91.343, 33.0844)
  line L270 (91.343, 41.9836) -> (91.343, 38.8844)
  line L271 (90.542, 41.9836) -> (90.542, 42.984)
  line L272 (90.542, 28.9833) -> (90.542, 29.9838)
  line L273 (91.343, 38.8844) -> (91.343, 41.9836)
  line L274 (90.542, 29.9838) -> (91.343, 29.9838)
  line L275 (91.343, 33.0844) -> (91.343, 29.9838)
  line L276 (91.343, 29.9838) -> (90.542, 29.9838)
  line L277 (91.343, 29.9838) -> (91.343, 33.0844)
  line L278 (91.343, 38.8844) -> (90.542, 38.8844)
  line L279 (76.542, 38.8844) -> (76.542, 33.0844)
  line L280 (76.542, 29.9838) -> (76.542, 28.9833)
  line L281 (75.742, 33.0844) -> (76.542, 33.0844)
  line L282 (76.542, 29.9838) -> (75.742, 29.9838)
  line L283 (76.542, 28.9833) -> (76.542, 29.9838)
  line L284 (75.742, 38.8844) -> (75.742, 41.9836)
  line L285 (76.542, 38.8844) -> (75.742, 38.8844)
  line L286 (76.542, 33.0844) -> (75.742, 33.0844)
  line L287 (75.742, 41.9836) -> (76.542, 41.9836)
  line L288 (90.542, 29.9838) -> (90.542, 28.9833)
  line L289 (76.542, 42.984) -> (76.542, 41.9836)
  line L290 (72.293, 29.9838) -> (72.293, 33.0844)
  line L291 (71.492, 42.984) -> (71.492, 41.9836)
  line L292 (72.293, 38.8844) -> (72.293, 41.9836)
  line L293 (71.492, 28.9833) -> (71.492, 29.9838)
  line L294 (71.492, 33.0844) -> (72.293, 33.0844)
  line L295 (71.492, 33.0844) -> (71.492, 38.8844)
  line L296 (72.293, 33.0844) -> (72.293, 29.9838)
  line L297 (72.293, 33.0844) -> (71.492, 33.0844)
  line L298 (72.293, 29.9838) -> (71.492, 29.9838)
  line L299 (72.293, 41.9836) -> (71.492, 41.9836)
  line L300 (71.492, 41.9836) -> (72.293, 41.9836)
  line L301 (72.293, 41.9836) -> (72.293, 38.8844)
  line L302 (71.492, 38.8844) -> (72.293, 38.8844)
  line L303 (71.492, 38.8844) -> (71.492, 33.0844)
  line L304 (71.492, 29.9838) -> (71.492, 28.9833)
  line L305 (71.492, 41.9836) -> (71.492, 42.984)
  line L306 (72.293, 38.8844) -> (71.492, 38.8844)
  line L307 (71.492, 29.9838) -> (72.293, 29.9838)
  line L308 (57.492, 41.9836) -> (57.492, 42.984)
  line L309 (97.687, 23.934) -> (83.685, 23.934)
  line L310 (83.685, 19.2336) -> (82.162, 19.2336)
  line L311 (83.685, 19.8345) -> (82.887, 19.8345)
  line L312 (83.685, 22.9336) -> (82.887, 22.9336)
  line L313 (80.435, 23.3844) -> (80.435, 22.4637)
  line L314 (74.587, 16.4335) -> (74.587, 19.2336)
  line L315 (74.587, 16.4335) -> (75.411, 16.4335)
  line L316 (80.435, 22.4637) -> (80.435, 23.3844)
  line L317 (77.137, 23.3844) -> (80.435, 23.3844)
  line L318 (77.137, 23.3844) -> (77.137, 22.4637)
  line L319 (82.887, 22.9336) -> (82.887, 19.8345)
  line L320 (74.587, 19.2336) -> (75.411, 19.2336)
  line L321 (82.162, 22.4637) -> (82.162, 19.2336)
  line L322 (77.137, 22.4637) -> (77.137, 23.3844)
  line L323 (80.435, 22.4637) -> (82.162, 22.4637)
  line L324 (82.162, 19.2336) -> (82.162, 22.4637)
  line L325 (83.685, 23.934) -> (83.685, 22.9336)
  line L326 (82.162, 19.2336) -> (83.685, 19.2336)
  line L327 (74.587, 19.2336) -> (74.587, 16.4335)
  line L328 (82.887, 22.9336) -> (83.685, 22.9336)
  line L329 (77.137, 22.4637) -> (75.411, 22.4637)
  line L330 (75.411, 19.2336) -> (74.587, 19.2336)
  line L331 (75.411, 19.2336) -> (75.411, 22.4637)
  line L332 (82.887, 19.8345) -> (83.685, 19.8345)
  line L333 (75.411, 22.4637) -> (75.411, 19.2336)
  line L334 (82.162, 22.4637) -> (80.435, 22.4637)
  line L335 (75.411, 22.4637) -> (77.137, 22.4637)
  line L336 (83.685, 23.934) -> (97.687, 23.934)
  line L337 (83.685, 19.8345) -> (83.685, 19.2336)
  line L338 (83.685, 19.2336) -> (83.685, 19.8345)
  line L339 (57.492, 42.984) -> (57.492, 41.9836)
  line L340 (62.768, 22.9336) -> (62.768, 19.8345)
  line L341 (61.967, 19.8345) -> (61.967, 14.0343)
  line L342 (62.768, 19.8345) -> (61.967, 19.8345)
  line L343 (61.967, 23.934) -> (47.967, 23.934)
  line L344 (47.967, 19.8345) -> (47.167, 19.8345)
  line L345 (47.167, 22.9336) -> (47.967, 22.9336)
  line L346 (47.967, 23.934) -> (47.967, 22.9336)
  line L347 (47.167, 22.9336) -> (47.167, 19.8345)
  line L348 (61.967, 14.0343) -> (61.967, 19.8345)
  line L349 (47.967, 19.8345) -> (47.967, 14.0343)
  line L350 (61.967, 23.934) -> (61.967, 22.9336)
  line L351 (47.967, 14.0343) -> (47.967, 19.8345)
  line L352 (61.967, 22.9336) -> (62.768, 22.9336)
  line L353 (62.768, 19.8345) -> (62.768, 22.9336)
  line L354 (57.492, 33.0844) -> (56.692, 33.0844)
  line L355 (56.692, 33.0844) -> (57.492, 33.0844)
  line L356 (53.243, 33.0844) -> (53.243, 29.9838)
  line L357 (52.442, 29.9838) -> (53.243, 29.9838)
  line L358 (53.243, 38.8844) -> (52.442, 38.8844)
  line L359 (53.243, 41.9836) -> (53.243, 38.8844)
  line L360 (52.442, 42.984) -> (38.442, 42.984)
  line L361 (52.442, 33.0844) -> (53.243, 33.0844)
  line L362 (57.492, 29.9838) -> (56.692, 29.9838)
  line L363 (53.243, 29.9838) -> (53.243, 33.0844)
  line L364 (57.492, 33.0844) -> (57.492, 38.8844)
  line L365 (52.442, 28.9833) -> (52.442, 29.9838)
  line L366 (52.442, 41.9836) -> (52.442, 42.984)
  line L367 (53.243, 33.0844) -> (52.442, 33.0844)
  line L368 (57.492, 38.8844) -> (56.692, 38.8844)
  line L369 (56.692, 41.9836) -> (57.492, 41.9836)
  line L370 (56.692, 33.0844) -> (56.692, 29.9838)
  line L371 (56.692, 38.8844) -> (57.492, 38.8844)
  line L372 (52.442, 42.984) -> (52.442, 41.9836)
  line L373 (53.243, 29.9838) -> (52.442, 29.9838)
  line L374 (53.243, 41.9836) -> (52.442, 41.9836)
  line L375 (56.692, 29.9838) -> (56.692, 33.0844)
  line L376 (57.492, 41.9836) -> (56.692, 41.9836)
  line L377 (52.442, 33.0844) -> (52.442, 38.8844)
  line L378 (52.442, 38.8844) -> (53.243, 38.8844)
  line L379 (52.442, 38.8844) -> (52.442, 33.0844)
  line L380 (57.492, 29.9838) -> (57.492, 28.9833)
  line L381 (56.692, 29.9838) -> (57.492, 29.9838)
  line L382 (57.492, 42.984) -> (71.492, 42.984)
  line L383 (52.442, 29.9838) -> (52.442, 28.9833)
  line L384 (53.243, 38.8844) -> (53.243, 41.9836)
  line L385 (52.442, 41.9836) -> (53.243, 41.9836)
  line L386 (56.692, 41.9836) -> (56.692, 38.8844)
  line L387 (57.492, 38.8844) -> (57.492, 33.0844)
  line L388 (56.692, 38.8844) -> (56.692, 41.9836)
  line L389 (57.492, 28.9833) -> (57.492, 29.9838)
  line L390 (71.492, 42.984) -> (57.492, 42.984)
  line L391 (71.492, 28.9833) -> (57.492, 28.9833)
  line L392 (57.492, 28.9833) -> (71.492, 28.9833)
  line L393 (82.162, 14.6338) -> (83.685, 14.6338)
  line L394 (83.685, 9.9333) -> (83.685, 10.9337)
  line L395 (82.887, 14.0343) -> (83.685, 14.0343)
  line L396 (80.435, 10.1634) -> (80.435, 9.1836)
  line L397 (74.161, 0.7845) -> (73.362, 0.7845)
  line L398 (73.362, 0.7845) -> (73.362, 3.8837)
  line L399 (83.685, 10.9337) -> (82.887, 10.9337)
  line L400 (82.887, 14.0343) -> (82.887, 10.9337)
  line L401 (82.887, 10.9337) -> (83.685, 10.9337)
  line L402 (83.685, 14.0343) -> (82.887, 14.0343)
  line L403 (57.206, 109.6602) -> (43.205, 109.6602)
  line L404 (75.411, 10.1634) -> (77.137, 10.1634)
  line L405 (88.162, 4.8841) -> (74.161, 4.8841)
  line L406 (74.161, 4.8841) -> (88.162, 4.8841)
  line L407 (82.162, 10.1634) -> (80.435, 10.1634)
  line L408 (97.687, 9.9333) -> (83.685, 9.9333)